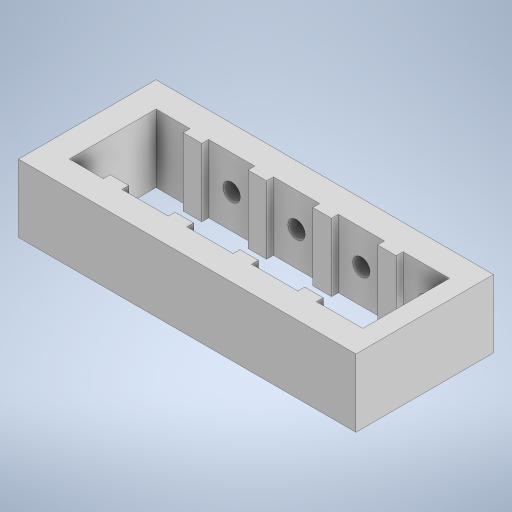
# Autodesk Inventor part: LatchBank
Saved by Autodesk Inventor 2024 (Build 280153000, 153)
## iProperties
Created: 2023-10-31
Part Number: LatchBank
Material: Generic
Document SubType Name: Modeling
Designer: gcter
Density: 1 g/cm^3
Appearance: Default
Author: gcter
Autodesk Inventor part; units mm, degrees
ref_plane "YZ Plane" through (0, 0, 0) normal (1, 0, 0) x (0, 1, 0)
ref_plane "XZ Plane" through (0, 0, 0) normal (0, 1, 0) x (-1, 0, 0)
ref_plane "XY Plane" through (0, 0, 0) normal (0, 0, 1) x (1, 0, 0)
sketch "Sketch1" plane through (0, 0, 0) normal (0, 1, 0) x (-1, 0, 0)
  line L0 (0, 0) -> (-5.08, 0)
  line L1 (-3.81, -3.81) -> (-3.81, -16.764)
  line L2 (-3.81, -20.574) -> (0, -20.574)
  line L3 (0, -20.574) -> (0, 0)
  line L4 (-3.81, -20.574) -> (-10.6172, -20.574)
  line L5 (-8.89, -16.764) -> (-3.81, -16.764)
  line L6 (-3.81, -3.81) -> (-8.89, -3.81)
  line L7 (-11.684, -16.764) -> (-11.684, -15.748)
  line L8 (-11.684, -15.748) -> (-8.89, -15.748)
  line L9 (-8.89, -15.748) -> (-8.89, -16.764)
  line L10 (-11.684, -3.81) -> (-11.684, -4.826)
  line L11 (-11.684, -4.826) -> (-8.89, -4.826)
  line L12 (-8.89, -4.826) -> (-8.89, -3.81)
  line L13 (-10.6172, -20.574) -> (-11.684, -20.574)
  line L14 (-11.684, -20.574) -> (-11.684, -16.764)
  line L15 (-5.08, 0) -> (-11.684, 0)
  line L16 (-11.684, 0) -> (-11.684, -3.81)
  point P0 (-1.905, -20.574)
  point P1 (-2.54, 0)
  point P2 (-3.81, -9.144)
  point P3 (-8.89, -16.256)
  point P4 (-11.684, -16.256)
  dimension "d1" = 20.574
  dimension "d4" = 3.81
  dimension "d6" = 5.08
  dimension "d7" = 3.81
  dimension "d8" = 2.794
  dimension "d11" = 1.016
  dimension "d12" = 1.016
  dimension "d28" = 3.81
  constraints: 34 end point, 5 horizontal, 5 parallel, 4 collinear, 4 midpoint, 2 perpendicular, 1 point on line
  measures "d1" distance from line of point (-2.54, 0) L2
  measures "d4" distance between parallel lines of L5 L4
  measures "d6" distance between parallel lines of L1 L9
  measures "d7" distance between parallel lines of L3 L1
  measures "d8" distance from line of point (-8.89, -16.256) L7
  measures "d11" distance between parallel lines of L5 L8
  measures "d12" distance between parallel lines of L6 L11
  measures "d28" distance between parallel lines of L15 L6
extrude "Extrusion1" add sketch "Sketch1" along normal blind 10.16
sketch "Sketch2" plane through (0, 0, 0) normal (0, -1, 0) x (1, 0, 0)
  line L0 (0, 0) -> (11.684, 0) projected
  line L1 (11.684, 0) -> (18.5928, 0)
  line L2 (18.5928, -3.81) -> (11.684, -3.81)
  line L3 (11.684, -3.81) -> (11.684, 0)
  line L4 (8.89, -3.81) -> (3.81, -3.81) projected
  line L5 (8.89, -4.826) -> (8.89, -3.81) projected
  line L6 (3.81, -3.81) -> (3.81, -16.764) projected
  line L7 (18.5928, 0) -> (21.3868, 0)
  line L8 (21.3868, 0) -> (21.3868, -4.826)
  line L9 (21.3868, -4.826) -> (18.5928, -4.826)
  line L10 (18.5928, -4.826) -> (18.5928, -3.81)
  line L11 (11.684, -4.826) -> (8.89, -4.826) projected
  line L12 (11.684, 0) -> (11.684, -4.826) projected
  line L13 (11.684, -16.764) -> (18.5928, -16.764)
  line L14 (23.0335, -20.574) -> (11.684, -20.574)
  line L15 (11.684, -20.574) -> (11.684, -16.764)
  line L16 (18.5928, -15.748) -> (21.3868, -15.748)
  line L17 (21.3868, -15.748) -> (21.3868, -20.574)
  line L18 (21.3868, -20.574) -> (23.0335, -20.574)
  line L19 (18.5928, -16.764) -> (18.5928, -15.748)
  line L20 (11.684, -20.574) -> (0, -20.574) projected
  line L21 (8.89, -15.748) -> (11.684, -15.748) projected
  line L22 (3.81, -16.764) -> (8.89, -16.764) projected
  point P0 (18.5928, -4.318)
  dimension "d32" = 2.794
  dimension "d33" = 6.9088
  constraints: 28 end point, 9 collinear, 6 parallel, 4 horizontal, 2 perpendicular, 1 midpoint
  measures "d32" distance from line of L8 point (18.593, -4.318)
  measures "d33" distance between parallel lines of L12 L10
extrude "Extrusion2" add sketch "Sketch2" against normal blind 10.16
sketch "Sketch3" plane through (11.684, 0, -16.764) normal (0, 0, 1) x (1, 0, 0)
  line L0 (6.9088, 0) -> (6.9088, 10.16) construction
  line L1 (0, 0) -> (0, 10.16) construction
  line L2 (0, 10.16) -> (6.9088, 10.16) construction
  line L3 (6.9088, 0) -> (0, 0) construction
  line L4 (6.9088, 10.16) -> (0, 0) construction
  line L5 (0, 10.16) -> (6.9088, 0) construction
  circle A0 centre (3.4544, 5.08) radius 1.3
  point P0 (-11.684, 0)
  dimension "d39" = 2.6
  constraints: 4 end point, 1 centre point, 1 midpoint
  measures "d39" diameter of A0
extrude "Extrusion3" cut sketch "Sketch3" against normal blind 10.16
pattern_linear "Rectangular Pattern2" count 4 spacing 9.7028 along (1, 0, 0) of "Extrusion2", "Extrusion3"
sketch "Sketch4" plane through (50.4952, 0, 0) normal (1, 0, 0) x (0, 0, -1)
  line L0 (20.574, 10.16) -> (0, 10.16) projected
  line L1 (20.574, 0) -> (0, 0) projected
  line L2 (0, 10.16) -> (20.574, 10.16)
  line L3 (20.574, 10.16) -> (20.574, 0)
  line L4 (20.574, 0) -> (0, 0)
  line L5 (0, 0) -> (0, 10.16)
  constraints: 8 end point, 2 parallel, 1 horizontal, 1 perpendicular
extrude "Extrusion4" add sketch "Sketch4" against normal blind 2.794
body "Solid1"
